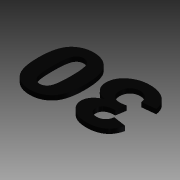
# Autodesk Inventor part: 30
Saved by Autodesk Inventor 2014 (Build 180170000, 170)
## iProperties
Created: 2017-08-29
Part Number: 30
Material: Generic
Document SubType Name: Modeling
Designer: resaj
Density: 1 g/cm^3
Appearance: Smooth - Black
Author: resaj
Autodesk Inventor part; units mm, degrees
ref_plane "YZ Plane" through (0, 0, 0) normal (1, 0, 0) x (0, 1, 0)
ref_plane "XZ Plane" through (0, 0, 0) normal (0, 1, 0) x (-1, 0, 0)
ref_plane "XY Plane" through (0, 0, 0) normal (0, 0, 1) x (1, 0, 0)
sketch "Sketch1" plane through (0, 0, 0) normal (0, 1, 0) x (-1, 0, 0)
  line L0 (-15.9712, 9.1405) -> (15.5875, 9.1405) construction
  line L1 (15.5875, 9.1405) -> (15.5875, -9.9475) construction
  line L2 (15.5875, -9.9475) -> (-15.9712, -9.9475) construction
  line L3 (-15.9712, -9.9475) -> (-15.9712, 9.1405) construction
  line L4 (-14.8909, -4.1596) -> (-11.0608, -3.7528)
  spline S0 degree 2 poles (-11.0608, -3.7528) (-10.9065, -5.0154) (-9.251, -6.3623) (-8.1146, -6.3623) knots 0 0 0 1 2 2 2
  spline S1 degree 2 poles (-8.1146, -6.3623) (-6.894, -6.3623) (-5.1965, -4.7629) (-5.1965, -3.3599) knots 0 0 0 1 2 2 2
  spline S2 degree 2 poles (-5.1965, -3.3599) (-5.1965, -2.0552) (-6.8239, -0.554) (-7.9884, -0.554) knots 0 0 0 1 2 2 2
  spline S3 degree 2 poles (-7.9884, -0.554) (-8.746, -0.554) (-9.7982, -0.8065) knots 0 0 0 1 1 1
  line L5 (-9.7982, -0.8065) -> (-9.3633, 1.9994)
  spline S4 degree 2 poles (-9.3633, 1.9994) (-7.82, 1.9713) (-6.9221, 2.5886) knots 0 0 0 1 1 1
  spline S5 degree 2 poles (-6.9221, 2.5886) (-6.0382, 3.2059) (-6.0382, 4.3143) knots 0 0 0 1 1 1
  spline S6 degree 2 poles (-6.0382, 4.3143) (-6.0382, 5.2543) (-7.329, 6.3065) (-8.3251, 6.3065) knots 0 0 0 1 2 2 2
  spline S7 degree 2 poles (-8.3251, 6.3065) (-9.3352, 6.3065) (-10.8083, 5.0859) (-10.9486, 3.8934) knots 0 0 0 1 2 2 2
  line L6 (-10.9486, 3.8934) -> (-14.6103, 4.4405)
  spline S8 degree 2 poles (-14.6103, 4.4405) (-14.0351, 6.9098) (-10.7241, 9.1405) (-8.2128, 9.1405) knots 0 0 0 1 2 2 2
  spline S9 degree 2 poles (-8.2128, 9.1405) (-5.3788, 9.1405) (-2.0538, 6.2644) (-2.0538, 4.5247) knots 0 0 0 1 2 2 2
  spline S10 degree 2 poles (-2.0538, 4.5247) (-2.0538, 3.3462) (-3.541, 1.4522) (-5.0421, 0.7508) knots 0 0 0 1 2 2 2
  spline S11 degree 2 poles (-5.0421, 0.7508) (-3.3025, 0.414) (-1.1279, -1.8447) (-1.1279, -3.5283) knots 0 0 0 1 2 2 2
  spline S12 degree 2 poles (-1.1279, -3.5283) (-1.1279, -5.9975) (-5.2386, -9.2243) (-8.0866, -9.2243) knots 0 0 0 1 2 2 2
  spline S13 degree 2 poles (-8.0866, -9.2243) (-10.8083, -9.2243) (-14.5823, -6.5026) (-14.8909, -4.1596) knots 0 0 0 1 2 2 2
  spline S14 degree 2 poles (8.0194, 9.1405) (11.0218, 9.1405) (14.7396, 5.0578) (14.7396, -0.0489) knots 0 0 0 1 2 2 2
  spline S15 degree 2 poles (14.7396, -0.0489) (14.7396, -5.1417) (11.0218, -9.2243) (8.0335, -9.2243) knots 0 0 0 1 2 2 2
  spline S16 degree 2 poles (8.0335, -9.2243) (5.0311, -9.2243) (1.3133, -5.1697) (1.3133, -0.0068) knots 0 0 0 1 2 2 2
  spline S17 degree 2 poles (1.3133, -0.0068) (1.3133, 5.0578) (5.0311, 9.1405) (8.0194, 9.1405) knots 0 0 0 1 2 2 2
  spline S18 degree 2 poles (8.0194, 6.2784) (6.8409, 6.2784) (5.452, 4.0758) (5.452, -0.0489) knots 0 0 0 1 2 2 2
  spline S19 degree 2 poles (5.452, -0.0489) (5.452, -4.1736) (6.8409, -6.3623) (8.0194, -6.3623) knots 0 0 0 1 2 2 2
  spline S20 degree 2 poles (8.0194, -6.3623) (9.1979, -6.3623) (10.5728, -4.1596) (10.5728, -0.0489) knots 0 0 0 1 2 2 2
  spline S21 degree 2 poles (10.5728, -0.0489) (10.5728, 4.0758) (9.1979, 6.2784) (8.0194, 6.2784) knots 0 0 0 1 2 2 2
  point P0 (0, 0)
  constraints: 2 other
extrude "Extrusion1" add sketch "Sketch1" along normal blind 1.3
body "Solid1"
